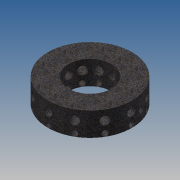
# Autodesk Inventor part: 2h4cem
Saved by Autodesk Inventor 2014 SP1 (Build 180222100, 222)
## iProperties
Company: HERA Project
Created: 2013-05-20
Part Number: 2h4cem
Material: Concrete
Document SubType Name: Modeling
Designer: David DeBoer
Density: 2.40731 g/cm^3
Description: Hub cement
Mass: 233879 g
Surface Area: 30868 cm^2
Volume: 97153.7 cm^3
Appearance: Exposed Aggregate - Coarse
Author: David DeBoer
Title: Cement
Autodesk Inventor part; units mm, degrees
ref_plane "YZ Plane" through (0, 0, 0) normal (1, 0, 0) x (0, 1, 0)
ref_plane "XZ Plane" through (0, 0, 0) normal (0, 1, 0) x (-1, 0, 0)
ref_plane "XY Plane" through (0, 0, 0) normal (0, 0, 1) x (1, 0, 0)
sketch "Sketch1" plane through (0, 0, 0) normal (0, 1, 0) x (-1, 0, 0)
  circle A0 centre (1.7415, 0) radius 450.85
  circle A1 centre (1.7415, 0) radius 229.87
  point P0 (0, 0)
  dimension "d0" = 901.7
  dimension "d4" = 459.74
  constraints: 2 centre point
  measures "d0" diameter of A0
  measures "d4" diameter of A1
extrude "Extrusion1" add sketch "Sketch1" along normal blind 254
sketch "Sketch2" plane through (-1.7415, 254, 0) normal (0, 1, 0) x (1, 0, 0)
  circle A0 centre (0, 0) radius 229.87 projected
  circle A1 centre (0, 0) radius 450.85 projected
  point P0 (1.7415, 0)
  point P1 (450.85, 0)
  constraints: 1 horizontal alignment, 1 other
ref_plane "Work Plane1" through (449.1085, 254, 0) normal (1, 0, 0) x (0, 1, 0)
sketch "Sketch5" plane through (-1.7415, 254, 0) normal (0, 1, 0) x (1, 0, 0)
  circle A0 centre (0, 0) radius 229.87 projected
  circle A1 centre (0, 0) radius 450.85 projected
  point P0 (1.7415, 0)
  point P1 (1.7415, 450.8466)
  constraints: 2 other
ref_plane "Work Plane2" through (0, 254, -450.8466) normal (0.0038627, 0, -0.9999925) x (-0.9999925, 0, -0.0038627)
sketch "Sketch6" plane through (0, 254, -450.8466) normal (0.0038627, 0, -0.9999925) x (-0.9999925, 0, -0.0038627)
  circle A0 centre (-1.7415, -104.14) radius 44.45
  line L0 (-450.85, -254) -> (450.85, -254) projected
  circle A1 centre (0, -223.52) radius 30.1625
  point P0 (-1.7415, -254)
  dimension "d15" = 88.9
  dimension "d17" = 149.86
  dimension "d18" = 60.325
  dimension "d19" = 30.48
  constraints: 2 centre point
  measures "d15" diameter of A0
  measures "d17" distance from line of A0.centre L0
  measures "d18" diameter of A1
  measures "d19" distance from line of L0 A1.centre
extrude "Extrusion4" cut sketch "Sketch6" against normal blind 254
pattern_circular "Circular Pattern1" count 12 over 360 about axis through (-1.7415, 0, 0) along (0, 1, 0) of "Extrusion4"
sketch "Sketch7" plane through (-1.7415, 254, 0) normal (0, 1, 0) x (1, 0, 0)
  circle A0 centre (0, 0) radius 229.87 projected
  circle A1 centre (0, 0) radius 450.85 projected
  line L0 (1.7415, 0) -> (492.4318, 131.4801) construction
  line L1 (1.7415, 0) -> (509.7415, 0) construction
  point P0 (435.6041, 116.2531)
  dimension "d25" = 508
  dimension "d26" = 15
  constraints: 4 end point, 1 horizontal, 1 point on line, 2 other
  measures "d25" distance of L0.start L0.end
  measures "d26" angle of L1 L0
ref_plane "Work Plane3" through (433.8626, 254, -116.2531) normal (0.9661841, 0, -0.2578532) x (0, 1, 0)
sketch "Sketch8" plane through (433.8626, 254, -116.2531) normal (0.9661841, 0, -0.2578532) x (0, 1, 0)
  circle A0 centre (-152.4, 0.4491) radius 30.1625
  line L0 (-254, 450.85) -> (-254, -450.85) projected
  point P0 (-254, 0.4491)
  dimension "d27" = 60.325
  dimension "d28" = 101.6
  constraints: 1 centre point
  measures "d27" diameter of A0
  measures "d28" distance from line of A0.centre L0
extrude "Extrusion5" cut sketch "Sketch8" against normal blind 254
body "Solid1"
